Autodesk Fusion 360 part; units mm, degrees
(part 3 of 6)
  spline S37 degree 5 poles (53.0142, 47.6687) (53.0234, 47.6622) (53.0419, 47.6493) (53.0695, 47.6299) (53.1065, 47.6042) (53.1527, 47.5723) (53.1991, 47.5406) (53.2455, 47.5092) (53.292, 47.478) (53.3386, 47.4471) (53.3852, 47.4164) (53.4319, 47.3859) (53.4787, 47.3557) (53.5256, 47.3258) (53.5726, 47.2961) (53.6196, 47.2667) (53.6667, 47.2375) (53.7139, 47.2086) (53.7612, 47.1799) (53.8085, 47.1515) (53.8559, 47.1233) (53.9034, 47.0955) (53.951, 47.0679) (53.9986, 47.0405) (54.0463, 47.0135) (54.0941, 46.9867) (54.142, 46.9602) (54.1899, 46.9339) (54.2379, 46.908) (54.286, 46.8823) (54.3341, 46.8569) (54.3823, 46.8318) (54.4306, 46.807) (54.4789, 46.7825) (54.5273, 46.7583) (54.5758, 46.7344) (54.6244, 46.7108) (54.673, 46.6875) (54.7217, 46.6646) (54.7704, 46.6419) (54.8193, 46.6196) (54.8682, 46.5976) (54.9171, 46.5759) (54.9662, 46.5546) (55.0152, 46.5336) (55.0644, 46.5129) (55.1136, 46.4926) (55.1629, 46.4726) (55.2123, 46.453) (55.2617, 46.4338) (55.3112, 46.4149) (55.3607, 46.3965) (55.4103, 46.3784) (55.46, 46.3608) (55.5098, 46.3436) (55.5596, 46.3268) (55.6095, 46.3104) (55.6594, 46.2943) (55.7094, 46.2787) (55.7594, 46.2635) (55.8095, 46.2488) (55.8597, 46.2348) (55.91, 46.2215) (55.9604, 46.2089) (56.0108, 46.1968) (56.0613, 46.1852) (56.1118, 46.1739) (56.1624, 46.163) (56.213, 46.1525) (56.2636, 46.143) (56.3144, 46.1348) (56.3552, 46.1299) (56.3859, 46.1272) (56.4064, 46.126) (56.4167, 46.1255) knots -1 -1 -1 -1 -1 -1 -0.98571429 -0.97142857 -0.95714286 -0.94285714 -0.92857143 -0.91428571 -0.9 -0.88571429 -0.87142857 -0.85714286 -0.84285714 -0.82857143 -0.81428571 -0.8 -0.78571429 -0.77142857 -0.75714286 -0.74285714 -0.72857143 -0.71428571 -0.7 -0.68571429 -0.67142857 -0.65714286 -0.64285714 -0.62857143 -0.61428571 -0.6 -0.58571429 -0.57142857 -0.55714286 -0.54285714 -0.52857143 -0.51428571 -0.5 -0.48571429 -0.47142857 -0.45714286 -0.44285714 -0.42857143 -0.41428571 -0.4 -0.38571429 -0.37142857 -0.35714286 -0.34285714 -0.32857143 -0.31428571 -0.3 -0.28571429 -0.27142857 -0.25714286 -0.24285714 -0.22857143 -0.21428571 -0.2 -0.18571429 -0.17142857 -0.15714286 -0.14285714 -0.12857143 -0.11428571 -0.1 -0.08571429 -0.07142857 -0.05714286 -0.04285714 -0.02857143 -0.01428571 0 0 0 0 0 0
  line L37 (56.4167, 46.1255) -> (56.9142, 46.1012)
  arc A75 (57.3897, 45.5888) -> (56.9142, 46.1012) centre (56.8899, 45.6018) ccw
  arc A76 (57.3897, 45.5888) -> (57.3897, 44.4112) centre (79.882, 45) ccw
  arc A77 (56.9142, 43.8988) -> (57.3897, 44.4112) centre (56.8899, 44.3982) ccw
  line L38 (56.9142, 43.8988) -> (56.4167, 43.8745)
  spline S38 degree 5 poles (56.4167, 43.8745) (56.4064, 43.874) (56.3859, 43.8728) (56.3552, 43.8701) (56.3144, 43.8652) (56.2636, 43.857) (56.213, 43.8475) (56.1624, 43.837) (56.1118, 43.8261) (56.0613, 43.8148) (56.0108, 43.8032) (55.9604, 43.7911) (55.91, 43.7785) (55.8597, 43.7652) (55.8095, 43.7512) (55.7594, 43.7365) (55.7094, 43.7213) (55.6594, 43.7057) (55.6095, 43.6896) (55.5596, 43.6732) (55.5098, 43.6564) (55.46, 43.6392) (55.4103, 43.6216) (55.3607, 43.6035) (55.3112, 43.5851) (55.2617, 43.5662) (55.2123, 43.547) (55.1629, 43.5274) (55.1136, 43.5074) (55.0644, 43.4871) (55.0152, 43.4664) (54.9662, 43.4454) (54.9171, 43.4241) (54.8682, 43.4024) (54.8193, 43.3804) (54.7704, 43.3581) (54.7217, 43.3354) (54.673, 43.3125) (54.6244, 43.2892) (54.5758, 43.2656) (54.5273, 43.2417) (54.4789, 43.2175) (54.4306, 43.193) (54.3823, 43.1682) (54.3341, 43.1431) (54.286, 43.1177) (54.2379, 43.092) (54.1899, 43.0661) (54.142, 43.0398) (54.0941, 43.0133) (54.0463, 42.9865) (53.9986, 42.9595) (53.951, 42.9321) (53.9034, 42.9045) (53.8559, 42.8767) (53.8085, 42.8485) (53.7612, 42.8201) (53.7139, 42.7914) (53.6667, 42.7625) (53.6196, 42.7333) (53.5726, 42.7039) (53.5256, 42.6742) (53.4787, 42.6443) (53.4319, 42.6141) (53.3852, 42.5836) (53.3386, 42.5529) (53.292, 42.522) (53.2455, 42.4908) (53.1991, 42.4594) (53.1527, 42.4277) (53.1065, 42.3958) (53.0695, 42.3701) (53.0419, 42.3507) (53.0234, 42.3378) (53.0142, 42.3313) knots 0 0 0 0 0 0 0.01428571 0.02857143 0.04285714 0.05714286 0.07142857 0.08571429 0.1 0.11428571 0.12857143 0.14285714 0.15714286 0.17142857 0.18571429 0.2 0.21428571 0.22857143 0.24285714 0.25714286 0.27142857 0.28571429 0.3 0.31428571 0.32857143 0.34285714 0.35714286 0.37142857 0.38571429 0.4 0.41428571 0.42857143 0.44285714 0.45714286 0.47142857 0.48571429 0.5 0.51428571 0.52857143 0.54285714 0.55714286 0.57142857 0.58571429 0.6 0.61428571 0.62857143 0.64285714 0.65714286 0.67142857 0.68571429 0.7 0.71428571 0.72857143 0.74285714 0.75714286 0.77142857 0.78571429 0.8 0.81428571 0.82857143 0.84285714 0.85714286 0.87142857 0.88571429 0.9 0.91428571 0.92857143 0.94285714 0.95714286 0.97142857 0.98571429 1 1 1 1 1 1
  arc A78 (53.0142, 42.3313) -> (53.1946, 40.9031) centre (79.882, 45) ccw
  spline S39 degree 5 poles (53.1946, 40.9031) (53.2052, 40.8991) (53.2263, 40.8912) (53.2579, 40.8793) (53.3001, 40.8635) (53.3528, 40.8441) (53.4055, 40.825) (53.4583, 40.8061) (53.5111, 40.7875) (53.5639, 40.7691) (53.6167, 40.751) (53.6696, 40.7331) (53.7224, 40.7155) (53.7753, 40.6982) (53.8281, 40.6811) (53.881, 40.6643) (53.9339, 40.6477) (53.9868, 40.6314) (54.0397, 40.6154) (54.0926, 40.5997) (54.1455, 40.5842) (54.1985, 40.569) (54.2514, 40.5541) (54.3043, 40.5395) (54.3573, 40.5251) (54.4102, 40.5111) (54.4632, 40.4973) (54.5161, 40.4838) (54.569, 40.4706) (54.622, 40.4577) (54.6749, 40.4451) (54.7279, 40.4328) (54.7808, 40.4207) (54.8337, 40.409) (54.8866, 40.3976) (54.9395, 40.3865) (54.9924, 40.3758) (55.0453, 40.3653) (55.0982, 40.3552) (55.151, 40.3453) (55.2039, 40.3358) (55.2567, 40.3267) (55.3095, 40.3179) (55.3623, 40.3094) (55.4151, 40.3013) (55.4679, 40.2935) (55.5206, 40.2861) (55.5733, 40.279) (55.626, 40.2723) (55.6786, 40.2659) (55.7312, 40.2599) (55.7838, 40.2544) (55.8364, 40.2493) (55.8889, 40.2446) (55.9413, 40.2403) (55.9938, 40.2364) (56.0461, 40.2329) (56.0985, 40.2297) (56.1508, 40.227) (56.2031, 40.2247) (56.2552, 40.223) (56.3073, 40.2219) (56.3594, 40.2215) (56.4113, 40.2218) (56.4632, 40.2227) (56.5149, 40.224) (56.5667, 40.2256) (56.6183, 40.2276) (56.6699, 40.2301) (56.7214, 40.2334) (56.7726, 40.2381) (56.8133, 40.2435) (56.8437, 40.2486) (56.8639, 40.2525) (56.874, 40.2545) knots -1 -1 -1 -1 -1 -1 -0.98571429 -0.97142857 -0.95714286 -0.94285714 -0.92857143 -0.91428571 -0.9 -0.88571429 -0.87142857 -0.85714286 -0.84285714 -0.82857143 -0.81428571 -0.8 -0.78571429 -0.77142857 -0.75714286 -0.74285714 -0.72857143 -0.71428571 -0.7 -0.68571429 -0.67142857 -0.65714286 -0.64285714 -0.62857143 -0.61428571 -0.6 -0.58571429 -0.57142857 -0.55714286 -0.54285714 -0.52857143 -0.51428571 -0.5 -0.48571429 -0.47142857 -0.45714286 -0.44285714 -0.42857143 -0.41428571 -0.4 -0.38571429 -0.37142857 -0.35714286 -0.34285714 -0.32857143 -0.31428571 -0.3 -0.28571429 -0.27142857 -0.25714286 -0.24285714 -0.22857143 -0.21428571 -0.2 -0.18571429 -0.17142857 -0.15714286 -0.14285714 -0.12857143 -0.11428571 -0.1 -0.08571429 -0.07142857 -0.05714286 -0.04285714 -0.02857143 -0.01428571 0 0 0 0 0 0
  line L39 (56.874, 40.2545) -> (57.3619, 40.3548)
  arc A79 (57.9499, 39.9767) -> (57.3619, 40.3548) centre (57.4626, 39.865) ccw
  arc A80 (57.9499, 39.9767) -> (58.2428, 38.8361) centre (79.882, 45) ccw
  arc A81 (57.9097, 38.2215) -> (58.2428, 38.8361) centre (57.7619, 38.6992) ccw
  line L40 (57.9097, 38.2215) -> (57.4338, 38.0743)
  spline S40 degree 5 poles (57.4338, 38.0743) (57.424, 38.0712) (57.4044, 38.0649) (57.3753, 38.0547) (57.337, 38.0398) (57.2899, 38.0193) (57.2432, 37.9974) (57.1968, 37.9747) (57.1506, 37.9515) (57.1044, 37.9281) (57.0584, 37.9043) (57.0126, 37.88) (56.9669, 37.8553) (56.9215, 37.8299) (56.8764, 37.8038) (56.8315, 37.7772) (56.7868, 37.75) (56.7423, 37.7224) (56.6979, 37.6944) (56.6537, 37.6661) (56.6096, 37.6375) (56.5657, 37.6084) (56.522, 37.579) (56.4784, 37.5492) (56.435, 37.519) (56.3917, 37.4884) (56.3487, 37.4575) (56.3057, 37.4262) (56.263, 37.3946) (56.2203, 37.3627) (56.1779, 37.3305) (56.1355, 37.298) (56.0934, 37.2651) (56.0513, 37.2319) (56.0094, 37.1985) (55.9677, 37.1647) (55.9261, 37.1306) (55.8847, 37.0962) (55.8434, 37.0616) (55.8022, 37.0267) (55.7612, 36.9915) (55.7203, 36.956) (55.6796, 36.9202) (55.639, 36.8842) (55.5985, 36.8479) (55.5582, 36.8114) (55.518, 36.7745) (55.478, 36.7375) (55.4381, 36.7001) (55.3984, 36.6626) (55.3587, 36.6247) (55.3193, 36.5866) (55.2799, 36.5483) (55.2407, 36.5097) (55.2017, 36.4709) (55.1627, 36.4319) (55.1239, 36.3926) (55.0853, 36.3531) (55.0468, 36.3133) (55.0084, 36.2734) (54.9702, 36.2331) (54.9321, 36.1927) (54.8941, 36.152) (54.8563, 36.1112) (54.8186, 36.07) (54.781, 36.0287) (54.7436, 35.9872) (54.7063, 35.9454) (54.6692, 35.9034) (54.6322, 35.8613) (54.5953, 35.8189) (54.5659, 35.7848) (54.544, 35.7591) (54.5293, 35.7419) (54.522, 35.7334) knots 0 0 0 0 0 0 0.01428571 0.02857143 0.04285714 0.05714286 0.07142857 0.08571429 0.1 0.11428571 0.12857143 0.14285714 0.15714286 0.17142857 0.18571429 0.2 0.21428571 0.22857143 0.24285714 0.25714286 0.27142857 0.28571429 0.3 0.31428571 0.32857143 0.34285714 0.35714286 0.37142857 0.38571429 0.4 0.41428571 0.42857143 0.44285714 0.45714286 0.47142857 0.48571429 0.5 0.51428571 0.52857143 0.54285714 0.55714286 0.57142857 0.58571429 0.6 0.61428571 0.62857143 0.64285714 0.65714286 0.67142857 0.68571429 0.7 0.71428571 0.72857143 0.74285714 0.75714286 0.77142857 0.78571429 0.8 0.81428571 0.82857143 0.84285714 0.85714286 0.87142857 0.88571429 0.9 0.91428571 0.92857143 0.94285714 0.95714286 0.97142857 0.98571429 1 1 1 1 1 1
  arc A82 (54.522, 35.7334) -> (55.0519, 34.395) centre (79.882, 45) ccw
  spline S41 degree 5 poles (55.0519, 34.395) (55.0631, 34.3937) (55.0855, 34.3912) (55.1191, 34.3876) (55.1639, 34.3828) (55.2198, 34.3772) (55.2756, 34.3717) (55.3314, 34.3666) (55.3872, 34.3616) (55.4429, 34.357) (55.4986, 34.3526) (55.5542, 34.3484) (55.6098, 34.3445) (55.6653, 34.3408) (55.7207, 34.3374) (55.7761, 34.3343) (55.8315, 34.3314) (55.8868, 34.3288) (55.942, 34.3265) (55.9972, 34.3244) (56.0523, 34.3225) (56.1073, 34.321) (56.1623, 34.3197) (56.2172, 34.3187) (56.272, 34.318) (56.3268, 34.3175) (56.3815, 34.3173) (56.4362, 34.3174) (56.4907, 34.3178) (56.5452, 34.3185) (56.5996, 34.3194) (56.654, 34.3207) (56.7082, 34.3222) (56.7624, 34.324) (56.8165, 34.3261) (56.8705, 34.3285) (56.9244, 34.3313) (56.9782, 34.3343) (57.0319, 34.3376) (57.0856, 34.3412) (57.1391, 34.3452) (57.1926, 34.3494) (57.2459, 34.354) (57.2992, 34.359) (57.3523, 34.3642) (57.4053, 34.3698) (57.4582, 34.3757) (57.5111, 34.382) (57.5638, 34.3886) (57.6163, 34.3955) (57.6688, 34.4028) (57.7211, 34.4105) (57.7733, 34.4186) (57.8253, 34.4271) (57.8772, 34.436) (57.9289, 34.4453) (57.9805, 34.4549) (58.032, 34.4649) (58.0834, 34.4752) (58.1345, 34.486) (58.1855, 34.4974) (58.2362, 34.5093) (58.2867, 34.5218) (58.337, 34.535) (58.387, 34.5487) (58.4368, 34.5629) (58.4865, 34.5773) (58.5361, 34.5921) (58.5854, 34.6073) (58.6344, 34.6233) (58.6829, 34.6407) (58.721, 34.656) (58.7491, 34.6685) (58.7677, 34.6773) (58.777, 34.6818) knots -1 -1 -1 -1 -1 -1 -0.98571429 -0.97142857 -0.95714286 -0.94285714 -0.92857143 -0.91428571 -0.9 -0.88571429 -0.87142857 -0.85714286 -0.84285714 -0.82857143 -0.81428571 -0.8 -0.78571429 -0.77142857 -0.75714286 -0.74285714 -0.72857143 -0.71428571 -0.7 -0.68571429 -0.67142857 -0.65714286 -0.64285714 -0.62857143 -0.61428571 -0.6 -0.58571429 -0.57142857 -0.55714286 -0.54285714 -0.52857143 -0.51428571 -0.5 -0.48571429 -0.47142857 -0.45714286 -0.44285714 -0.42857143 -0.41428571 -0.4 -0.38571429 -0.37142857 -0.35714286 -0.34285714 -0.32857143 -0.31428571 -0.3 -0.28571429 -0.27142857 -0.25714286 -0.24285714 -0.22857143 -0.21428571 -0.2 -0.18571429 -0.17142857 -0.15714286 -0.14285714 -0.12857143 -0.11428571 -0.1 -0.08571429 -0.07142857 -0.05714286 -0.04285714 -0.02857143 -0.01428571 0 0 0 0 0 0
  line L41 (58.777, 34.6818) -> (59.2247, 34.9002)
  arc A83 (59.8882, 34.6802) -> (59.2247, 34.9002) centre (59.4439, 34.4509) ccw
  arc A84 (59.8882, 34.6802) -> (60.4555, 33.6483) centre (79.882, 45) ccw
  arc A85 (60.2857, 32.9702) -> (60.4555, 33.6483) centre (60.0238, 33.3961) ccw
  line L42 (60.2857, 32.9702) -> (59.8614, 32.7092)
  spline S42 degree 5 poles (59.8614, 32.7092) (59.8526, 32.7038) (59.8353, 32.6928) (59.8096, 32.6757) (59.7763, 32.6518) (59.7357, 32.6202) (59.6959, 32.5874) (59.6566, 32.5538) (59.6176, 32.5199) (59.5788, 32.4857) (59.5401, 32.4512) (59.5017, 32.4163) (59.4637, 32.381) (59.426, 32.3451) (59.3888, 32.3086) (59.3519, 32.2717) (59.3154, 32.2342) (59.2791, 32.1964) (59.2431, 32.1583) (59.2073, 32.1199) (59.1718, 32.0812) (59.1364, 32.0421) (59.1014, 32.0028) (59.0666, 31.9631) (59.0321, 31.923) (58.9978, 31.8826) (58.9638, 31.842) (58.93, 31.801) (58.8964, 31.7598) (58.863, 31.7182) (58.8299, 31.6765) (58.797, 31.6344) (58.7643, 31.5921) (58.7318, 31.5495) (58.6996, 31.5067) (58.6676, 31.4636) (58.6358, 31.4202) (58.6042, 31.3767) (58.5728, 31.3328) (58.5416, 31.2888) (58.5106, 31.2445) (58.4799, 31.1999) (58.4493, 31.1552) (58.4189, 31.1102) (58.3888, 31.065) (58.3588, 31.0195) (58.3291, 30.9739) (58.2995, 30.928) (58.2702, 30.8819) (58.241, 30.8356) (58.212, 30.7892) (58.1833, 30.7425) (58.1547, 30.6955) (58.1263, 30.6484) (58.0981, 30.6011) (58.0701, 30.5536) (58.0423, 30.5059) (58.0147, 30.4581) (57.9873, 30.41) (57.9601, 30.3617) (57.933, 30.3132) (57.9062, 30.2646) (57.8795, 30.2158) (57.8531, 30.1668) (57.8268, 30.1176) (57.8007, 30.0682) (57.7748, 30.0187) (57.7491, 29.9689) (57.7235, 29.9191) (57.6982, 29.869) (57.673, 29.8187) (57.653, 29.7784) (57.6381, 29.7481) (57.6282, 29.7278) (57.6233, 29.7177) knots 0 0 0 0 0 0 0.01428571 0.02857143 0.04285714 0.05714286 0.07142857 0.08571429 0.1 0.11428571 0.12857143 0.14285714 0.15714286 0.17142857 0.18571429 0.2 0.21428571 0.22857143 0.24285714 0.25714286 0.27142857 0.28571429 0.3 0.31428571 0.32857143 0.34285714 0.35714286 0.37142857 0.38571429 0.4 0.41428571 0.42857143 0.44285714 0.45714286 0.47142857 0.48571429 0.5 0.51428571 0.52857143 0.54285714 0.55714286 0.57142857 0.58571429 0.6 0.61428571 0.62857143 0.64285714 0.65714286 0.67142857 0.68571429 0.7 0.71428571 0.72857143 0.74285714 0.75714286 0.77142857 0.78571429 0.8 0.81428571 0.82857143 0.84285714 0.85714286 0.87142857 0.88571429 0.9 0.91428571 0.92857143 0.94285714 0.95714286 0.97142857 0.98571429 1 1 1 1 1 1
  arc A86 (57.6233, 29.7177) -> (58.4694, 28.5532) centre (79.882, 45) ccw
  spline S43 degree 5 poles (58.4694, 28.5532) (58.4805, 28.5547) (58.5028, 28.5579) (58.5363, 28.5627) (58.5808, 28.5692) (58.6364, 28.5776) (58.6918, 28.5863) (58.7472, 28.5952) (58.8024, 28.6043) (58.8575, 28.6136) (58.9125, 28.6231) (58.9675, 28.6329) (59.0222, 28.643) (59.0769, 28.6532) (59.1315, 28.6637) (59.1859, 28.6745) (59.2402, 28.6855) (59.2944, 28.6967) (59.3485, 28.7081) (59.4025, 28.7198) (59.4563, 28.7318) (59.51, 28.744) (59.5636, 28.7564) (59.617, 28.7691) (59.6703, 28.782) (59.7235, 28.7952) (59.7765, 28.8086) (59.8294, 28.8223) (59.8822, 28.8362) (59.9348, 28.8504) (59.9872, 28.8649) (60.0395, 28.8796) (60.0917, 28.8946) (60.1437, 28.9098) (60.1956, 28.9253) (60.2473, 28.9411) (60.2988, 28.9571) (60.3502, 28.9734) (60.4015, 28.99) (60.4525, 29.0069) (60.5034, 29.024) (60.5541, 29.0414) (60.6046, 29.0591) (60.655, 29.0771) (60.7051, 29.0955) (60.7551, 29.1141) (60.8049, 29.1329) (60.8545, 29.1521) (60.9039, 29.1716) (60.9531, 29.1914) (61.0021, 29.2115) (61.0508, 29.232) (61.0993, 29.2528) (61.1476, 29.274) (61.1957, 29.2955) (61.2435, 29.3174) (61.2911, 29.3395) (61.3384, 29.362) (61.3856, 29.3848) (61.4325, 29.408) (61.479, 29.4316) (61.5252, 29.4558) (61.571, 29.4805) (61.6164, 29.5057) (61.6614, 29.5315) (61.7061, 29.5576) (61.7507, 29.5839) (61.795, 29.6106) (61.839, 29.6376) (61.8825, 29.6653) (61.9251, 29.6941) (61.9582, 29.7184) (61.9824, 29.7375) (61.9982, 29.7507) (62.0061, 29.7573) knots -1 -1 -1 -1 -1 -1 -0.98571429 -0.97142857 -0.95714286 -0.94285714 -0.92857143 -0.91428571 -0.9 -0.88571429 -0.87142857 -0.85714286 -0.84285714 -0.82857143 -0.81428571 -0.8 -0.78571429 -0.77142857 -0.75714286 -0.74285714 -0.72857143 -0.71428571 -0.7 -0.68571429 -0.67142857 -0.65714286 -0.64285714 -0.62857143 -0.61428571 -0.6 -0.58571429 -0.57142857 -0.55714286 -0.54285714 -0.52857143 -0.51428571 -0.5 -0.48571429 -0.47142857 -0.45714286 -0.44285714 -0.42857143 -0.41428571 -0.4 -0.38571429 -0.37142857 -0.35714286 -0.34285714 -0.32857143 -0.31428571 -0.3 -0.28571429 -0.27142857 -0.25714286 -0.24285714 -0.22857143 -0.21428571 -0.2 -0.18571429 -0.17142857 -0.15714286 -0.14285714 -0.12857143 -0.11428571 -0.1 -0.08571429 -0.07142857 -0.05714286 -0.04285714 -0.02857143 -0.01428571 0 0 0 0 0 0
  line L43 (62.0061, 29.7573) -> (62.3854, 30.0802)
  arc A87 (63.0828, 30.0321) -> (62.3854, 30.0802) centre (62.7095, 29.6995) ccw
  arc A88 (63.0828, 30.0321) -> (63.8889, 29.1738) centre (79.882, 45) ccw
  arc A89 (63.8931, 28.4747) -> (63.8889, 29.1738) centre (63.5335, 28.8221) ccw
  line L44 (63.8931, 28.4747) -> (63.547, 28.1164)
  spline S44 degree 5 poles (63.547, 28.1164) (63.5398, 28.109) (63.5257, 28.0941) (63.5052, 28.0711) (63.4788, 28.0396) (63.4473, 27.9989) (63.417, 27.9573) (63.3873, 27.915) (63.3579, 27.8724) (63.3288, 27.8296) (63.2999, 27.7866) (63.2714, 27.7433) (63.2434, 27.6996) (63.2158, 27.6555) (63.1888, 27.6109) (63.1623, 27.5659) (63.1362, 27.5206) (63.1105, 27.4749) (63.0851, 27.4291) (63.06, 27.3829) (63.0352, 27.3366) (63.0107, 27.29) (62.9865, 27.2432) (62.9627, 27.196) (62.9392, 27.1487) (62.9161, 27.101) (62.8932, 27.0532) (62.8707, 27.0051) (62.8484, 26.9568) (62.8264, 26.9083) (62.8047, 26.8596) (62.7833, 26.8107) (62.7622, 26.7616) (62.7413, 26.7123) (62.7207, 26.6628) (62.7004, 26.613) (62.6804, 26.5632) (62.6606, 26.5131) (62.6411, 26.4628) (62.6219, 26.4124) (62.6029, 26.3618) (62.5842, 26.311) (62.5657, 26.26) (62.5475, 26.2089) (62.5295, 26.1576) (62.5118, 26.1062) (62.4943, 26.0545) (62.4771, 26.0028) (62.4601, 25.9508) (62.4434, 25.8987) (62.4269, 25.8465) (62.4107, 25.7941) (62.3947, 25.7416) (62.3789, 25.6889) (62.3634, 25.6361) (62.3481, 25.5831) (62.333, 25.53) (62.3182, 25.4767) (62.3036, 25.4234) (62.2892, 25.3698) (62.2751, 25.3162) (62.2612, 25.2624) (62.2475, 25.2085) (62.234, 25.1544) (62.2208, 25.1002) (62.2078, 25.0459) (62.195, 24.9915) (62.1825, 24.9369) (62.1701, 24.8823) (62.158, 24.8275) (62.1462, 24.7725) (62.1368, 24.7285) (62.1299, 24.6954) (62.1254, 24.6734) (62.1231, 24.6623) knots 0 0 0 0 0 0 0.01428571 0.02857143 0.04285714 0.05714286 0.07142857 0.08571429 0.1 0.11428571 0.12857143 0.14285714 0.15714286 0.17142857 0.18571429 0.2 0.21428571 0.22857143 0.24285714 0.25714286 0.27142857 0.28571429 0.3 0.31428571 0.32857143 0.34285714 0.35714286 0.37142857 0.38571429 0.4 0.41428571 0.42857143 0.44285714 0.45714286 0.47142857 0.48571429 0.5 0.51428571 0.52857143 0.54285714 0.55714286 0.57142857 0.58571429 0.6 0.61428571 0.62857143 0.64285714 0.65714286 0.67142857 0.68571429 0.7 0.71428571 0.72857143 0.74285714 0.75714286 0.77142857 0.78571429 0.8 0.81428571 0.82857143 0.84285714 0.85714286 0.87142857 0.88571429 0.9 0.91428571 0.92857143 0.94285714 0.95714286 0.97142857 0.98571429 1 1 1 1 1 1
  arc A90 (62.1231, 24.6623) -> (63.2322, 23.7448) centre (79.882, 45) ccw
  spline S45 degree 5 poles (63.2322, 23.7448) (63.2427, 23.7491) (63.2635, 23.7577) (63.2947, 23.7706) (63.3362, 23.788) (63.3879, 23.81) (63.4395, 23.8322) (63.4909, 23.8545) (63.5421, 23.8771) (63.5932, 23.8998) (63.6441, 23.9228) (63.6948, 23.9459) (63.7454, 23.9692) (63.7958, 23.9928) (63.8461, 24.0165) (63.8961, 24.0405) (63.946, 24.0646) (63.9957, 24.089) (64.0452, 24.1135) (64.0946, 24.1383) (64.1437, 24.1632) (64.1927, 24.1884) (64.2415, 24.2137) (64.2901, 24.2393) (64.3385, 24.2651) (64.3868, 24.2911) (64.4348, 24.3173) (64.4826, 24.3437) (64.5303, 24.3703) (64.5777, 24.3971) (64.6249, 24.4242) (64.6719, 24.4514) (64.7187, 24.4789) (64.7653, 24.5066) (64.8117, 24.5345) (64.8579, 24.5626) (64.9038, 24.591) (64.9495, 24.6196) (64.995, 24.6484) (65.0403, 24.6774) (65.0853, 24.7066) (65.1301, 24.7361) (65.1746, 24.7659) (65.2189, 24.7958) (65.2629, 24.826) (65.3067, 24.8565) (65.3502, 24.8871) (65.3935, 24.9181) (65.4365, 24.9492) (65.4792, 24.9806) (65.5216, 25.0123) (65.5638, 25.0442) (65.6056, 25.0765) (65.6471, 25.109) (65.6883, 25.1418) (65.7291, 25.1748) (65.7697, 25.2081) (65.81, 25.2417) (65.85, 25.2755) (65.8897, 25.3096) (65.9289, 25.3441) (65.9676, 25.379) (66.0058, 25.4143) (66.0435, 25.45) (66.0807, 25.4862) (66.1175, 25.5226) (66.1541, 25.5592) (66.1905, 25.596) (66.2264, 25.6331) (66.2616, 25.6707) (66.2957, 25.7093) (66.3217, 25.7411) (66.3404, 25.7656) (66.3524, 25.7822) (66.3584, 25.7906) knots -1 -1 -1 -1 -1 -1 -0.98571429 -0.97142857 -0.95714286 -0.94285714 -0.92857143 -0.91428571 -0.9 -0.88571429 -0.87142857 -0.85714286 -0.84285714 -0.82857143 -0.81428571 -0.8 -0.78571429 -0.77142857 -0.75714286 -0.74285714 -0.72857143 -0.71428571 -0.7 -0.68571429 -0.67142857 -0.65714286 -0.64285714 -0.62857143 -0.61428571 -0.6 -0.58571429 -0.57142857 -0.55714286 -0.54285714 -0.52857143 -0.51428571 -0.5 -0.48571429 -0.47142857 -0.45714286 -0.44285714 -0.42857143 -0.41428571 -0.4 -0.38571429 -0.37142857 -0.35714286 -0.34285714 -0.32857143 -0.31428571 -0.3 -0.28571429 -0.27142857 -0.25714286 -0.24285714 -0.22857143 -0.21428571 -0.2 -0.18571429 -0.17142857 -0.15714286 -0.14285714 -0.12857143 -0.11428571 -0.1 -0.08571429 -0.07142857 -0.05714286 -0.04285714 -0.02857143 -0.01428571 0 0 0 0 0 0
  line L45 (66.3584, 25.7906) -> (66.6454, 26.1977)
  arc A91 (67.3329, 26.3246) -> (66.6454, 26.1977) centre (67.0541, 25.9096) ccw
  arc A92 (67.3329, 26.3246) -> (68.3271, 25.6937) centre (79.882, 45) ccw
  arc A93 (68.5051, 25.0176) -> (68.3271, 25.6937) centre (68.0704, 25.2646) ccw
  line L46 (68.5051, 25.0176) -> (68.2589, 24.5845)
  spline S46 degree 5 poles (68.2589, 24.5845) (68.2539, 24.5755) (68.2439, 24.5576) (68.2297, 24.5302) (68.212, 24.4931) (68.1917, 24.4459) (68.1726, 24.398) (68.1543, 24.3497) (68.1365, 24.3011) (68.1189, 24.2525) (68.1017, 24.2036) (68.0848, 24.1546) (68.0685, 24.1053) (68.0528, 24.0557) (68.0378, 24.0058) (68.0233, 23.9556) (68.0093, 23.9052) (67.9957, 23.8546) (67.9825, 23.8039) (67.9697, 23.753) (67.9572, 23.7019) (67.945, 23.6507) (67.9333, 23.5993) (67.9219, 23.5477) (67.9109, 23.496) (67.9004, 23.4441) (67.8901, 23.3921) (67.8803, 23.3399) (67.8707, 23.2876) (67.8615, 23.2351) (67.8526, 23.1826) (67.844, 23.1299) (67.8357, 23.077) (67.8278, 23.0241) (67.8202, 22.971) (67.8129, 22.9178) (67.8059, 22.8645) (67.7992, 22.8111) (67.7928, 22.7576) (67.7867, 22.7039) (67.7809, 22.6502) (67.7754, 22.5963) (67.7702, 22.5424) (67.7652, 22.4883) (67.7606, 22.4342) (67.7562, 22.3799) (67.7522, 22.3256) (67.7484, 22.2712) (67.7448, 22.2167) (67.7416, 22.162) (67.7386, 22.1073) (67.7359, 22.0526) (67.7334, 21.9977) (67.7313, 21.9427) (67.7294, 21.8877) (67.7277, 21.8326) (67.7263, 21.7774) (67.7252, 21.7221) (67.7243, 21.6668) (67.7237, 21.6114) (67.7234, 21.5559) (67.7233, 21.5003) (67.7235, 21.4447) (67.7239, 21.389) (67.7245, 21.3332) (67.7254, 21.2774) (67.7266, 21.2215) (67.728, 21.1656) (67.7297, 21.1095) (67.7316, 21.0534) (67.7337, 20.9973) (67.7356, 20.9523) (67.7372, 20.9186) (67.7383, 20.8961) (67.7388, 20.8848) knots 0 0 0 0 0 0 0.01428571 0.02857143 0.04285714 0.05714286 0.07142857 0.08571429 0.1 0.11428571 0.12857143 0.14285714 0.15714286 0.17142857 0.18571429 0.2 0.21428571 0.22857143 0.24285714 0.25714286 0.27142857 0.28571429 0.3 0.31428571 0.32857143 0.34285714 0.35714286 0.37142857 0.38571429 0.4 0.41428571 0.42857143 0.44285714 0.45714286 0.47142857 0.48571429 0.5 0.51428571 0.52857143 0.54285714 0.55714286 0.57142857 0.58571429 0.6 0.61428571 0.62857143 0.64285714 0.65714286 0.67142857 0.68571429 0.7 0.71428571 0.72857143 0.74285714 0.75714286 0.77142857 0.78571429 0.8 0.81428571 0.82857143 0.84285714 0.85714286 0.87142857 0.88571429 0.9 0.91428571 0.92857143 0.94285714 0.95714286 0.97142857 0.98571429 1 1 1 1 1 1
  arc A94 (67.7388, 20.8848) -> (69.0413, 20.2719) centre (79.882, 45) ccw
  spline S47 degree 5 poles (69.0413, 20.2719) (69.0503, 20.2787) (69.0684, 20.2922) (69.0954, 20.3125) (69.1312, 20.3397) (69.1759, 20.3738) (69.2203, 20.4081) (69.2645, 20.4425) (69.3085, 20.4771) (69.3523, 20.5119) (69.3959, 20.5467) (69.4393, 20.5818) (69.4825, 20.617) (69.5255, 20.6523) (69.5682, 20.6878) (69.6108, 20.7234) (69.6531, 20.7592) (69.6952, 20.7952) (69.737, 20.8312) (69.7787, 20.8675) (69.8201, 20.9039) (69.8613, 20.9404) (69.9022, 20.9771) (69.943, 21.014) (69.9834, 21.051) (70.0237, 21.0882) (70.0637, 21.1255) (70.1034, 21.163) (70.143, 21.2006) (70.1822, 21.2384) (70.2212, 21.2763) (70.26, 21.3144) (70.2985, 21.3526) (70.3367, 21.3911) (70.3747, 21.4296) (70.4124, 21.4683) (70.4499, 21.5072) (70.487, 21.5463) (70.5239, 21.5855) (70.5606, 21.6249) (70.5969, 21.6644) (70.6329, 21.7041) (70.6687, 21.744) (70.7041, 21.784) (70.7392, 21.8242) (70.7741, 21.8646) (70.8086, 21.9051) (70.8428, 21.9458) (70.8767, 21.9867) (70.9103, 22.0277) (70.9435, 22.069) (70.9764, 22.1104) (71.0089, 22.152) (71.041, 22.1938) (71.0727, 22.2358) (71.1041, 22.278) (71.1351, 22.3204) (71.1658, 22.3629) (71.1962, 22.4056) (71.2261, 22.4485) (71.2555, 22.4916) (71.2843, 22.535) (71.3125, 22.5787) (71.3401, 22.6227) (71.3672, 22.667) (71.3938, 22.7114) (71.4202, 22.756) (71.4462, 22.8007) (71.4718, 22.8455) (71.4965, 22.8908) (71.5199, 22.9365) (71.5372, 22.9738) (71.5492, 23.0022) (71.5568, 23.0213) (71.5604, 23.0309) knots -1 -1 -1 -1 -1 -1 -0.98571429 -0.97142857 -0.95714286 -0.94285714 -0.92857143 -0.91428571 -0.9 -0.88571429 -0.87142857 -0.85714286 -0.84285714 -0.82857143 -0.81428571 -0.8 -0.78571429 -0.77142857 -0.75714286 -0.74285714 -0.72857143 -0.71428571 -0.7 -0.68571429 -0.67142857 -0.65714286 -0.64285714 -0.62857143 -0.61428571 -0.6 -0.58571429 -0.57142857 -0.55714286 -0.54285714 -0.52857143 -0.51428571 -0.5 -0.48571429 -0.47142857 -0.45714286 -0.44285714 -0.42857143 -0.41428571 -0.4 -0.38571429 -0.37142857 -0.35714286 -0.34285714 -0.32857143 -0.31428571 -0.3 -0.28571429 -0.27142857 -0.25714286 -0.24285714 -0.22857143 -0.21428571 -0.2 -0.18571429 -0.17142857 -0.15714286 -0.14285714 -0.12857143 -0.11428571 -0.1 -0.08571429 -0.07142857 -0.05714286 -0.04285714 -0.02857143 -0.01428571 0 0 0 0 0 0
  line L47 (71.5604, 23.0309) -> (71.7372, 23.4966)
  arc A95 (72.3716, 23.7905) -> (71.7372, 23.4966) centre (72.2047, 23.3192) ccw
  arc A96 (72.3716, 23.7905) -> (73.4915, 23.4266) centre (79.882, 45) ccw
  arc A97 (73.8319, 22.816) -> (73.4915, 23.4266) centre (73.3494, 22.9472) ccw
  line L48 (73.8319, 22.816) -> (73.7012, 22.3353)
  spline S48 degree 5 poles (73.7012, 22.3353) (73.6985, 22.3254) (73.6934, 22.3055) (73.6864, 22.2755) (73.6785, 22.2352) (73.6705, 22.1844) (73.664, 22.1332) (73.6583, 22.0819) (73.6531, 22.0304) (73.6482, 21.9789) (73.6436, 21.9273) (73.6395, 21.8756) (73.636, 21.8238) (73.6331, 21.7719) (73.6309, 21.7198) (73.6294, 21.6676) (73.6283, 21.6153) (73.6278, 21.5629) (73.6276, 21.5105) (73.6278, 21.458) (73.6284, 21.4054) (73.6294, 21.3528) (73.6308, 21.3001) (73.6326, 21.2473) (73.6349, 21.1945) (73.6375, 21.1416) (73.6406, 21.0887) (73.644, 21.0357) (73.6477, 20.9826) (73.6518, 20.9295) (73.6563, 20.8764) (73.6611, 20.8232) (73.6662, 20.77) (73.6717, 20.7167) (73.6775, 20.6634) (73.6837, 20.6101) (73.6901, 20.5567) (73.697, 20.5033) (73.7041, 20.4499) (73.7115, 20.3964) (73.7193, 20.3429) (73.7273, 20.2894) (73.7357, 20.2358) (73.7443, 20.1823) (73.7533, 20.1287) (73.7626, 20.075) (73.7721, 20.0214) (73.782, 19.9677) (73.7921, 19.914) (73.8026, 19.8603) (73.8133, 19.8066) (73.8243, 19.7529) (73.8355, 19.6991) (73.8471, 19.6454) (73.8589, 19.5916) (73.8711, 19.5378) (73.8834, 19.484) (73.8961, 19.4302) (73.909, 19.3764) (73.9222, 19.3225) (73.9357, 19.2687) (73.9494, 19.2149) (73.9634, 19.161) (73.9776, 19.1072) (73.9922, 19.0533) (74.0069, 18.9995) (74.022, 18.9456) (74.0372, 18.8918) (74.0528, 18.8379) (74.0686, 18.7841) (74.0846, 18.7302) (74.0977, 18.6871) (74.1076, 18.6548) (74.1142, 18.6333) (74.1175, 18.6225) knots 0 0 0 0 0 0 0.01428571 0.02857143 0.04285714 0.05714286 0.07142857 0.08571429 0.1 0.11428571 0.12857143 0.14285714 0.15714286 0.17142857 0.18571429 0.2 0.21428571 0.22857143 0.24285714 0.25714286 0.27142857 0.28571429 0.3 0.31428571 0.32857143 0.34285714 0.35714286 0.37142857 0.38571429 0.4 0.41428571 0.42857143 0.44285714 0.45714286 0.47142857 0.48571429 0.5 0.51428571 0.52857143 0.54285714 0.55714286 0.57142857 0.58571429 0.6 0.61428571 0.62857143 0.64285714 0.65714286 0.67142857 0.68571429 0.7 0.71428571 0.72857143 0.74285714 0.75714286 0.77142857 0.78571429 0.8 0.81428571 0.82857143 0.84285714 0.85714286 0.87142857 0.88571429 0.9 0.91428571 0.92857143 0.94285714 0.95714286 0.97142857 0.98571429 1 1 1 1 1 1
  arc A98 (74.1175, 18.6225) -> (75.5315, 18.3528) centre (79.882, 45) ccw
  spline S49 degree 5 poles (75.5315, 18.3528) (75.5386, 18.3616) (75.5527, 18.3792) (75.5738, 18.4056) (75.6017, 18.4408) (75.6365, 18.485) (75.671, 18.5292) (75.7053, 18.5736) (75.7393, 18.618) (75.7731, 18.6626) (75.8067, 18.7072) (75.84, 18.7519) (75.8731, 18.7967) (75.9059, 18.8417) (75.9385, 18.8867) (75.9708, 18.9318) (76.0029, 18.9769) (76.0347, 19.0222) (76.0663, 19.0676) (76.0976, 19.1131) (76.1287, 19.1586) (76.1595, 19.2043) (76.19, 19.25) (76.2203, 19.2958) (76.2503, 19.3417) (76.28, 19.3877) (76.3095, 19.4338) (76.3387, 19.48) (76.3676, 19.5263) (76.3962, 19.5726) (76.4246, 19.6191) (76.4527, 19.6656) (76.4804, 19.7122) (76.5079, 19.759) (76.5351, 19.8058) (76.562, 19.8526) (76.5886, 19.8996) (76.6149, 19.9467) (76.6409, 19.9938) (76.6666, 20.0411) (76.6919, 20.0884) (76.717, 20.1358) (76.7417, 20.1833) (76.766, 20.2309) (76.7901, 20.2786) (76.8138, 20.3264) (76.8371, 20.3742) (76.8602, 20.4221) (76.8828, 20.4702) (76.9051, 20.5183) (76.9271, 20.5665) (76.9486, 20.6148) (76.9697, 20.6632) (76.9904, 20.7116) (77.0107, 20.7602) (77.0306, 20.8089) (77.0501, 20.8576) (77.0693, 20.9064) (77.0881, 20.9553) (77.1064, 21.0043) (77.1241, 21.0534) (77.1413, 21.1027) (77.1577, 21.152) (77.1735, 21.2015) (77.1887, 21.2511) (77.2034, 21.3007) (77.2179, 21.3504) (77.232, 21.4002) (77.2456, 21.45) (77.2583, 21.5) (77.2696, 21.5501) (77.2771, 21.5905) (77.2817, 21.621) (77.2842, 21.6414) (77.2853, 21.6516) knots -1 -1 -1 -1 -1 -1 -0.98571429 -0.97142857 -0.95714286 -0.94285714 -0.92857143 -0.91428571 -0.9 -0.88571429 -0.87142857 -0.85714286 -0.84285714 -0.82857143 -0.81428571 -0.8 -0.78571429 -0.77142857 -0.75714286 -0.74285714 -0.72857143 -0.71428571 -0.7 -0.68571429 -0.67142857 -0.65714286 -0.64285714 -0.62857143 -0.61428571 -0.6 -0.58571429 -0.57142857 -0.55714286 -0.54285714 -0.52857143 -0.51428571 -0.5 -0.48571429 -0.47142857 -0.45714286 -0.44285714 -0.42857143 -0.41428571 -0.4 -0.38571429 -0.37142857 -0.35714286 -0.34285714 -0.32857143 -0.31428571 -0.3 -0.28571429 -0.27142857 -0.25714286 -0.24285714 -0.22857143 -0.21428571 -0.2 -0.18571429 -0.17142857 -0.15714286 -0.14285714 -0.12857143 -0.11428571 -0.1 -0.08571429 -0.07142857 -0.05714286 -0.04285714 -0.02857143 -0.01428571 0 0 0 0 0 0
  line L49 (77.2853, 21.6516) -> (77.3408, 22.1467)
  arc A99 (77.8821, 22.5891) -> (77.3408, 22.1467) centre (77.8377, 22.091) ccw
  line L50 (79.882, 45) -> (99.5642, 63.4828) construction
  line L51 (94.2241, 62.3365) -> (103.1265, 70.6965)
  line L52 (106.9873, 66.5851) -> (98.0849, 58.2252)
  circle A100 centre (110.7338, 73.9718) radius 1.75
  arc A101 (111.7668, 69.0797) -> (105.9162, 75.3099) centre (110.7338, 73.9718) ccw
  arc A102 (103.1265, 70.6965) -> (105.9162, 75.3099) centre (96.281, 77.9862) ccw
  arc A103 (111.7668, 69.0797) -> (106.9873, 66.5851) centre (113.8328, 59.2954) ccw
  circle A104 centre (79.882, 45) radius 0.5
  circle A105 centre (79.882, 45) radius 1.75
  dimension "d193" = 3.5
  dimension "d194" = 10
  dimension "d195" = 10
  dimension "d1" = 3.5
  constraint coincident A0.centre A2.centre
  constraint midpoint A38 L50.end
  constraint midpoint A40 L51.start
  constraint midpoint A36 L52.end
  constraint parallel L50 L51
  constraint parallel L50 L52
  constraint concentric A100 A101
  constraint tangent L51 A102
  constraint tangent A101 A102
  constraint tangent A101 A103
  constraint tangent L52 A103
  constraint equal A102 A103
  measures "d193" diameter of A100
  measures "d194" diameter of A101
  measures "d195" radius of A102
  measures "d1" diameter of A105
extrude "Extruir4" add sketch "Boceto5" against normal up to surface (3 mm away) contours A36 A37 L18 S18 A38 S19 L19 A39 A40 L51 L52 A101 A102 A103
extrude "Extruir5" cut sketch "Boceto5" against normal up to surface (3 mm away) contours A105
sketch "Boceto6" plane through (3, 0, 0) normal (1, 0, 0) x (0, 1, 0)
  circle A0 centre (79.882, 45) radius 1.75
  circle A1 centre (110.7338, 73.9718) radius 1.75
  arc A2 (77.8821, 22.5891) -> (79.0573, 22.5151) centre (79.882, 45) ccw
  arc A3 (79.5389, 22.0084) -> (79.0573, 22.5151) centre (79.039, 22.0155) ccw
  line L0 (79.5389, 22.0084) -> (79.5319, 21.5103)
  spline S0 degree 5 poles (79.5319, 21.5103) (79.5317, 21.5) (79.5317, 21.4795) (79.5324, 21.4487) (79.5348, 21.4076) (79.5397, 21.3564) (79.5461, 21.3053) (79.5533, 21.2541) (79.5611, 21.203) (79.5692, 21.1519) (79.5776, 21.1008) (79.5864, 21.0497) (79.5959, 20.9986) (79.606, 20.9476) (79.6169, 20.8966) (79.6283, 20.8457) (79.6404, 20.7948) (79.6528, 20.7439) (79.6657, 20.6931) (79.679, 20.6423) (79.6926, 20.5915) (79.7067, 20.5408) (79.7211, 20.4901) (79.736, 20.4394) (79.7513, 20.3888) (79.767, 20.3382) (79.7831, 20.2877) (79.7996, 20.2372) (79.8165, 20.1868) (79.8336, 20.1364) (79.8512, 20.086) (79.869, 20.0357) (79.8872, 19.9854) (79.9058, 19.9352) (79.9247, 19.885) (79.9439, 19.8349) (79.9635, 19.7848) (79.9833, 19.7348) (80.0035, 19.6848) (80.024, 19.6348) (80.0448, 19.5849) (80.066, 19.5351) (80.0874, 19.4853) (80.1091, 19.4356) (80.1311, 19.3859) (80.1534, 19.3363) (80.176, 19.2867) (80.1989, 19.2371) (80.2221, 19.1877) (80.2455, 19.1382) (80.2693, 19.0889) (80.2933, 19.0396) (80.3176, 18.9903) (80.3421, 18.9411) (80.367, 18.892) (80.3921, 18.8429) (80.4175, 18.7938) (80.4431, 18.7449) (80.469, 18.696) (80.4952, 18.6471) (80.5216, 18.5983) (80.5483, 18.5496) (80.5752, 18.5009) (80.6024, 18.4523) (80.6299, 18.4038) (80.6576, 18.3553) (80.6855, 18.3068) (80.7137, 18.2585) (80.7422, 18.2102) (80.7709, 18.162) (80.7998, 18.1138) (80.8231, 18.0753) (80.8407, 18.0465) (80.8525, 18.0273) (80.8584, 18.0177) knots 0 0 0 0 0 0 0.01428571 0.02857143 0.04285714 0.05714286 0.07142857 0.08571429 0.1 0.11428571 0.12857143 0.14285714 0.15714286 0.17142857 0.18571429 0.2 0.21428571 0.22857143 0.24285714 0.25714286 0.27142857 0.28571429 0.3 0.31428571 0.32857143 0.34285714 0.35714286 0.37142857 0.38571429 0.4 0.41428571 0.42857143 0.44285714 0.45714286 0.47142857 0.48571429 0.5 0.51428571 0.52857143 0.54285714 0.55714286 0.57142857 0.58571429 0.6 0.61428571 0.62857143 0.64285714 0.65714286 0.67142857 0.68571429 0.7 0.71428571 0.72857143 0.74285714 0.75714286 0.77142857 0.78571429 0.8 0.81428571 0.82857143 0.84285714 0.85714286 0.87142857 0.88571429 0.9 0.91428571 0.92857143 0.94285714 0.95714286 0.97142857 0.98571429 1 1 1 1 1 1
  arc A4 (80.8584, 18.0177) -> (82.2951, 18.108) centre (79.882, 45) ccw
  spline S1 degree 5 poles (82.2951, 18.108) (82.2997, 18.1183) (82.309, 18.1388) (82.3229, 18.1697) (82.3412, 18.2108) (82.3639, 18.2622) (82.3863, 18.3136) (82.4085, 18.3651) (82.4304, 18.4166) (82.452, 18.4682) (82.4734, 18.5197) (82.4946, 18.5713) (82.5155, 18.623) (82.5361, 18.6746) (82.5565, 18.7263) (82.5766, 18.7781) (82.5964, 18.8298) (82.616, 18.8816) (82.6353, 18.9334) (82.6543, 18.9852) (82.6731, 19.037) (82.6916, 19.0889) (82.7098, 19.1408) (82.7277, 19.1927) (82.7453, 19.2447) (82.7627, 19.2966) (82.7798, 19.3486) (82.7966, 19.4006) (82.8131, 19.4526) (82.8293, 19.5046) (82.8452, 19.5566) (82.8608, 19.6087) (82.8761, 19.6608) (82.8911, 19.7129) (82.9058, 19.7649) (82.9202, 19.8171) (82.9343, 19.8692) (82.9481, 19.9213) (82.9615, 19.9734) (82.9746, 20.0256) (82.9874, 20.0777) (82.9999, 20.1299) (83.012, 20.182) (83.0238, 20.2342) (83.0352, 20.2863) (83.0462, 20.3385) (83.057, 20.3906) (83.0674, 20.4428) (83.0774, 20.495) (83.087, 20.5471) (83.0963, 20.5992) (83.1051, 20.6514) (83.1135, 20.7035) (83.1215, 20.7556) (83.1291, 20.8077) (83.1363, 20.8598) (83.1431, 20.9118) (83.1495, 20.9639) (83.1555, 21.0159) (83.161, 21.0679) (83.166, 21.1199) (83.1704, 21.1718) (83.174, 21.2237) (83.177, 21.2756) (83.1794, 21.3274) (83.1814, 21.3791) (83.183, 21.4309) (83.1842, 21.4826) (83.185, 21.5342) (83.1849, 21.5858) (83.1834, 21.6372) (83.1806, 21.6782) (83.1775, 21.7088) (83.1749, 21.7292) (83.1734, 21.7394) knots -1 -1 -1 -1 -1 -1 -0.98571429 -0.97142857 -0.95714286 -0.94285714 -0.92857143 -0.91428571 -0.9 -0.88571429 -0.87142857 -0.85714286 -0.84285714 -0.82857143 -0.81428571 -0.8 -0.78571429 -0.77142857 -0.75714286 -0.74285714 -0.72857143 -0.71428571 -0.7 -0.68571429 -0.67142857 -0.65714286 -0.64285714 -0.62857143 -0.61428571 -0.6 -0.58571429 -0.57142857 -0.55714286 -0.54285714 -0.52857143 -0.51428571 -0.5 -0.48571429 -0.47142857 -0.45714286 -0.44285714 -0.42857143 -0.41428571 -0.4 -0.38571429 -0.37142857 -0.35714286 -0.34285714 -0.32857143 -0.31428571 -0.3 -0.28571429 -0.27142857 -0.25714286 -0.24285714 -0.22857143 -0.21428571 -0.2 -0.18571429 -0.17142857 -0.15714286 -0.14285714 -0.12857143 -0.11428571 -0.1 -0.08571429 -0.07142857 -0.05714286 -0.04285714 -0.02857143 -0.01428571 0 0 0 0 0 0
  line L1 (83.1734, 21.7394) -> (83.104, 22.2327)
  arc A5 (83.5183, 22.7958) -> (83.104, 22.2327) centre (83.5991, 22.3024) ccw
  arc A6 (83.5183, 22.7958) -> (84.675, 23.0164) centre (79.882, 45) ccw
  arc A7 (85.2675, 22.6454) -> (84.675, 23.0164) centre (84.7815, 22.5279) ccw
  line L2 (85.2675, 22.6454) -> (85.3845, 22.1612)
  spline S2 degree 5 poles (85.3845, 22.1612) (85.387, 22.1512) (85.392, 22.1313) (85.4004, 22.1016) (85.4129, 22.0625) (85.4304, 22.0141) (85.4493, 21.9661) (85.469, 21.9184) (85.4892, 21.8708) (85.5098, 21.8233) (85.5306, 21.7759) (85.5519, 21.7286) (85.5738, 21.6815) (85.5963, 21.6346) (85.6195, 21.5879) (85.6432, 21.5414) (85.6675, 21.4951) (85.6923, 21.449) (85.7174, 21.4029) (85.7429, 21.357) (85.7687, 21.3112) (85.7949, 21.2656) (85.8216, 21.2201) (85.8486, 21.1747) (85.876, 21.1295) (85.9038, 21.0844) (85.932, 21.0395) (85.9605, 20.9947) (85.9893, 20.95) (86.0185, 20.9055) (86.048, 20.8611) (86.0778, 20.8168) (86.108, 20.7726) (86.1384, 20.7286) (86.1692, 20.6847) (86.2003, 20.6409) (86.2317, 20.5972) (86.2634, 20.5537) (86.2954, 20.5103) (86.3276, 20.467) (86.3602, 20.4239) (86.393, 20.3809) (86.4262, 20.338) (86.4596, 20.2952) (86.4932, 20.2525) (86.5272, 20.21) (86.5614, 20.1676) (86.5959, 20.1253) (86.6307, 20.0832) (86.6657, 20.0411) (86.7009, 19.9992) (86.7365, 19.9574) (86.7722, 19.9158) (86.8083, 19.8742) (86.8446, 19.8328) (86.8811, 19.7915) (86.9179, 19.7503) (86.9549, 19.7093) (86.9921, 19.6683) (87.0296, 19.6275) (87.0673, 19.5868) (87.1053, 19.5463) (87.1435, 19.5058) (87.1819, 19.4655) (87.2206, 19.4253) (87.2595, 19.3852) (87.2986, 19.3453) (87.3379, 19.3055) (87.3775, 19.2657) (87.4173, 19.2262) (87.4573, 19.1867) (87.4895, 19.1552) (87.5137, 19.1317) (87.5299, 19.116) (87.538, 19.1082) knots 0 0 0 0 0 0 0.01428571 0.02857143 0.04285714 0.05714286 0.07142857 0.08571429 0.1 0.11428571 0.12857143 0.14285714 0.15714286 0.17142857 0.18571429 0.2 0.21428571 0.22857143 0.24285714 0.25714286 0.27142857 0.28571429 0.3 0.31428571 0.32857143 0.34285714 0.35714286 0.37142857 0.38571429 0.4 0.41428571 0.42857143 0.44285714 0.45714286 0.47142857 0.48571429 0.5 0.51428571 0.52857143 0.54285714 0.55714286 0.57142857 0.58571429 0.6 0.61428571 0.62857143 0.64285714 0.65714286 0.67142857 0.68571429 0.7 0.71428571 0.72857143 0.74285714 0.75714286 0.77142857 0.78571429 0.8 0.81428571 0.82857143 0.84285714 0.85714286 0.87142857 0.88571429 0.9 0.91428571 0.92857143 0.94285714 0.95714286 0.97142857 0.98571429 1 1 1 1 1 1
  arc A8 (87.538, 19.1082) -> (88.907, 19.553) centre (79.882, 45) ccw
  spline S3 degree 5 poles (88.907, 19.553) (88.909, 19.5641) (88.9129, 19.5863) (88.9186, 19.6196) (88.9262, 19.664) (88.9353, 19.7194) (88.9443, 19.7748) (88.9529, 19.8302) (88.9613, 19.8855) (88.9695, 19.9408) (88.9774, 19.9961) (88.9851, 20.0514) (88.9924, 20.1066) (88.9996, 20.1618) (89.0064, 20.2169) (89.0131, 20.272) (89.0194, 20.327) (89.0255, 20.382) (89.0313, 20.437) (89.0368, 20.4919) (89.0421, 20.5468) (89.0471, 20.6017) (89.0518, 20.6565) (89.0563, 20.7112) (89.0605, 20.7659) (89.0644, 20.8205) (89.068, 20.8751) (89.0713, 20.9296) (89.0744, 20.9841) (89.0771, 21.0385) (89.0796, 21.0929) (89.0818, 21.1472) (89.0837, 21.2015) (89.0852, 21.2556) (89.0865, 21.3097) (89.0875, 21.3638) (89.0882, 21.4178) (89.0886, 21.4717) (89.0886, 21.5255) (89.0884, 21.5793) (89.0878, 21.633) (89.0869, 21.6866) (89.0856, 21.7401) (89.0841, 21.7936) (89.0822, 21.8469) (89.0799, 21.9002) (89.0773, 21.9534) (89.0744, 22.0065) (89.0711, 22.0595) (89.0675, 22.1124) (89.0635, 22.1652) (89.0591, 22.2179) (89.0543, 22.2705) (89.0491, 22.3229) (89.0435, 22.3753) (89.0375, 22.4275) (89.0311, 22.4796) (89.0244, 22.5316) (89.0173, 22.5835) (89.0097, 22.6353) (89.0016, 22.6868) (88.9929, 22.7382) (88.9835, 22.7894) (88.9735, 22.8404) (88.963, 22.8911) (88.952, 22.9418) (88.9407, 22.9923) (88.929, 23.0427) (88.917, 23.0929) (88.9041, 23.1428) (88.8898, 23.1922) (88.8769, 23.2312) (88.8662, 23.2601) (88.8586, 23.2792) (88.8547, 23.2887) knots -1 -1 -1 -1 -1 -1 -0.98571429 -0.97142857 -0.95714286 -0.94285714 -0.92857143 -0.91428571 -0.9 -0.88571429 -0.87142857 -0.85714286 -0.84285714 -0.82857143 -0.81428571 -0.8 -0.78571429 -0.77142857 -0.75714286 -0.74285714 -0.72857143 -0.71428571 -0.7 -0.68571429 -0.67142857 -0.65714286 -0.64285714 -0.62857143 -0.61428571 -0.6 -0.58571429 -0.57142857 -0.55714286 -0.54285714 -0.52857143 -0.51428571 -0.5 -0.48571429 -0.47142857 -0.45714286 -0.44285714 -0.42857143 -0.41428571 -0.4 -0.38571429 -0.37142857 -0.35714286 -0.34285714 -0.32857143 -0.31428571 -0.3 -0.28571429 -0.27142857 -0.25714286 -0.24285714 -0.22857143 -0.21428571 -0.2 -0.18571429 -0.17142857 -0.15714286 -0.14285714 -0.12857143 -0.11428571 -0.1 -0.08571429 -0.07142857 -0.05714286 -0.04285714 -0.02857143 -0.01428571 0 0 0 0 0 0
  line L3 (88.8547, 23.2887) -> (88.6648, 23.7492)
  arc A9 (88.926, 24.3977) -> (88.6648, 23.7492) centre (89.127, 23.9399) ccw
  arc A10 (88.926, 24.3977) -> (89.9915, 24.899) centre (79.882, 45) ccw
  arc A11 (90.6577, 24.687) -> (89.9915, 24.899) centre (90.2161, 24.4524) ccw
  line L4 (90.6577, 24.687) -> (90.8915, 24.2471)
  spline S4 degree 5 poles (90.8915, 24.2471) (90.8963, 24.2381) (90.9061, 24.22) (90.9216, 24.1934) (90.9434, 24.1586) (90.9724, 24.1161) (91.0027, 24.0743) (91.0336, 24.033) (91.0651, 23.9919) (91.0968, 23.951) (91.1288, 23.9103) (91.1612, 23.8698) (91.194, 23.8296) (91.2275, 23.7898) (91.2616, 23.7503) (91.2961, 23.7112) (91.3312, 23.6724) (91.3667, 23.6338) (91.4024, 23.5955) (91.4385, 23.5573) (91.4749, 23.5194) (91.5117, 23.4817) (91.5488, 23.4443) (91.5862, 23.4071) (91.624, 23.3701) (91.6622, 23.3333) (91.7006, 23.2968) (91.7394, 23.2605) (91.7784, 23.2244) (91.8178, 23.1885) (91.8574, 23.1528) (91.8973, 23.1174) (91.9375, 23.0821) (91.9779, 23.047) (92.0186, 23.0121) (92.0596, 22.9775) (92.1009, 22.943) (92.1424, 22.9087) (92.1842, 22.8746) (92.2262, 22.8408) (92.2685, 22.8071) (92.311, 22.7736) (92.3538, 22.7402) (92.3968, 22.7071) (92.44, 22.6742) (92.4834, 22.6414) (92.5271, 22.6089) (92.5711, 22.5765) (92.6152, 22.5443) (92.6596, 22.5123) (92.7042, 22.4805) (92.749, 22.4488) (92.794, 22.4174) (92.8392, 22.3861) (92.8846, 22.355) (92.9303, 22.3241) (92.9761, 22.2933) (93.0222, 22.2628) (93.0685, 22.2324) (93.1149, 22.2022) (93.1616, 22.1722) (93.2085, 22.1423) (93.2555, 22.1126) (93.3028, 22.0831) (93.3502, 22.0538) (93.3978, 22.0247) (93.4457, 21.9957) (93.4937, 21.9669) (93.5419, 21.9383) (93.5902, 21.9098) (93.6388, 21.8816) (93.6778, 21.8591) (93.7071, 21.8423) (93.7267, 21.8312) (93.7365, 21.8256) knots 0 0 0 0 0 0 0.01428571 0.02857143 0.04285714 0.05714286 0.07142857 0.08571429 0.1 0.11428571 0.12857143 0.14285714 0.15714286 0.17142857 0.18571429 0.2 0.21428571 0.22857143 0.24285714 0.25714286 0.27142857 0.28571429 0.3 0.31428571 0.32857143 0.34285714 0.35714286 0.37142857 0.38571429 0.4 0.41428571 0.42857143 0.44285714 0.45714286 0.47142857 0.48571429 0.5 0.51428571 0.52857143 0.54285714 0.55714286 0.57142857 0.58571429 0.6 0.61428571 0.62857143 0.64285714 0.65714286 0.67142857 0.68571429 0.7 0.71428571 0.72857143 0.74285714 0.75714286 0.77142857 0.78571429 0.8 0.81428571 0.82857143 0.84285714 0.85714286 0.87142857 0.88571429 0.9 0.91428571 0.92857143 0.94285714 0.95714286 0.97142857 0.98571429 1 1 1 1 1 1
  arc A12 (93.7365, 21.8256) -> (94.9519, 22.5969) centre (79.882, 45) ccw
  spline S5 degree 5 poles (94.9519, 22.5969) (94.951, 22.6081) (94.9493, 22.6306) (94.9466, 22.6643) (94.9428, 22.7091) (94.9379, 22.7651) (94.9328, 22.821) (94.9274, 22.8768) (94.9218, 22.9325) (94.916, 22.9881) (94.9099, 23.0436) (94.9035, 23.099) (94.897, 23.1543) (94.8902, 23.2095) (94.8831, 23.2646) (94.8758, 23.3197) (94.8683, 23.3746) (94.8605, 23.4294) (94.8524, 23.484) (94.8441, 23.5386) (94.8356, 23.5931) (94.8268, 23.6475) (94.8178, 23.7017) (94.8085, 23.7558) (94.7989, 23.8098) (94.7891, 23.8637) (94.779, 23.9175) (94.7687, 23.9711) (94.7581, 24.0247) (94.7472, 24.0781) (94.7361, 24.1313) (94.7247, 24.1845) (94.713, 24.2375) (94.7011, 24.2904) (94.6889, 24.3431) (94.6764, 24.3957) (94.6636, 24.4481) (94.6506, 24.5004) (94.6372, 24.5526) (94.6236, 24.6046) (94.6097, 24.6565) (94.5955, 24.7082) (94.581, 24.7597) (94.5662, 24.8111) (94.5511, 24.8623) (94.5356, 24.9133) (94.5199, 24.9642) (94.5039, 25.0149) (94.4875, 25.0654) (94.4709, 25.1158) (94.4539, 25.1659) (94.4365, 25.2159) (94.4188, 25.2656) (94.4007, 25.3151) (94.3822, 25.3644) (94.3634, 25.4135) (94.3443, 25.4624) (94.3248, 25.5111) (94.305, 25.5596) (94.2848, 25.6078) (94.2642, 25.6558) (94.2429, 25.7034) (94.2212, 25.7506) (94.1988, 25.7975) (94.1759, 25.8441) (94.1527, 25.8904) (94.1292, 25.9365) (94.1054, 25.9824) (94.0812, 26.028) (94.0563, 26.0732) (94.0302, 26.1175) (94.008, 26.1521) (93.9905, 26.1774) (93.9783, 26.194) (93.9722, 26.2022) knots -1 -1 -1 -1 -1 -1 -0.98571429 -0.97142857 -0.95714286 -0.94285714 -0.92857143 -0.91428571 -0.9 -0.88571429 -0.87142857 -0.85714286 -0.84285714 -0.82857143 -0.81428571 -0.8 -0.78571429 -0.77142857 -0.75714286 -0.74285714 -0.72857143 -0.71428571 -0.7 -0.68571429 -0.67142857 -0.65714286 -0.64285714 -0.62857143 -0.61428571 -0.6 -0.58571429 -0.57142857 -0.55714286 -0.54285714 -0.52857143 -0.51428571 -0.5 -0.48571429 -0.47142857 -0.45714286 -0.44285714 -0.42857143 -0.41428571 -0.4 -0.38571429 -0.37142857 -0.35714286 -0.34285714 -0.32857143 -0.31428571 -0.3 -0.28571429 -0.27142857 -0.25714286 -0.24285714 -0.22857143 -0.21428571 -0.2 -0.18571429 -0.17142857 -0.15714286 -0.14285714 -0.12857143 -0.11428571 -0.1 -0.08571429 -0.07142857 -0.05714286 -0.04285714 -0.02857143 -0.01428571 0 0 0 0 0 0
  line L5 (93.9722, 26.2022) -> (93.6737, 26.6011)
  arc A13 (93.7655, 27.2941) -> (93.6737, 26.6011) centre (94.074, 26.9006) ccw
  arc A14 (93.7655, 27.2941) -> (94.6728, 28.0447) centre (79.882, 45) ccw
  arc A15 (95.3708, 28.005) -> (94.6728, 28.0447) centre (95.0015, 27.6679) ccw
  line L6 (95.3708, 28.005) -> (95.7066, 27.6371)
  spline S6 degree 5 poles (95.7066, 27.6371) (95.7135, 27.6295) (95.7276, 27.6145) (95.7492, 27.5925) (95.779, 27.5642) (95.8176, 27.5303) (95.8573, 27.4973) (95.8976, 27.465) (95.9382, 27.433) (95.9791, 27.4013) (96.0202, 27.3698) (96.0617, 27.3386) (96.1035, 27.3079) (96.1458, 27.2776) (96.1886, 27.2479) (96.2319, 27.2186) (96.2755, 27.1897) (96.3194, 27.1612) (96.3636, 27.1329) (96.408, 27.105) (96.4527, 27.0773) (96.4977, 27.0499) (96.5429, 27.0229) (96.5885, 26.9962) (96.6343, 26.9697) (96.6803, 26.9436) (96.7267, 26.9178) (96.7733, 26.8923) (96.8201, 26.8671) (96.8671, 26.8421) (96.9143, 26.8174) (96.9618, 26.7929) (97.0095, 26.7687) (97.0574, 26.7448) (97.1055, 26.7212) (97.1538, 26.6978) (97.2024, 26.6747) (97.2511, 26.6518) (97.3001, 26.6292) (97.3492, 26.6068) (97.3985, 26.5847) (97.448, 26.5628) (97.4977, 26.5412) (97.5476, 26.5198) (97.5977, 26.4986) (97.6479, 26.4777) (97.6983, 26.457) (97.7489, 26.4366) (97.7997, 26.4164) (97.8506, 26.3964) (97.9017, 26.3767) (97.953, 26.3572) (98.0044, 26.3379) (98.056, 26.3189) (98.1077, 26.3) (98.1596, 26.2814) (98.2117, 26.2631) (98.2639, 26.2449) (98.3163, 26.227) (98.3688, 26.2093) (98.4215, 26.1918) (98.4743, 26.1746) (98.5272, 26.1575) (98.5803, 26.1407) (98.6336, 26.1241) (98.687, 26.1077) (98.7405, 26.0916) (98.7941, 26.0756) (98.8479, 26.0599) (98.9019, 26.0444) (98.9559, 26.0291) (98.9993, 26.017) (99.0319, 26.008) (99.0536, 26.0021) (99.0645, 25.9991) knots 0 0 0 0 0 0 0.01428571 0.02857143 0.04285714 0.05714286 0.07142857 0.08571429 0.1 0.11428571 0.12857143 0.14285714 0.15714286 0.17142857 0.18571429 0.2 0.21428571 0.22857143 0.24285714 0.25714286 0.27142857 0.28571429 0.3 0.31428571 0.32857143 0.34285714 0.35714286 0.37142857 0.38571429 0.4 0.41428571 0.42857143 0.44285714 0.45714286 0.47142857 0.48571429 0.5 0.51428571 0.52857143 0.54285714 0.55714286 0.57142857 0.58571429 0.6 0.61428571 0.62857143 0.64285714 0.65714286 0.67142857 0.68571429 0.7 0.71428571 0.72857143 0.74285714 0.75714286 0.77142857 0.78571429 0.8 0.81428571 0.82857143 0.84285714 0.85714286 0.87142857 0.88571429 0.9 0.91428571 0.92857143 0.94285714 0.95714286 0.97142857 0.98571429 1 1 1 1 1 1
  arc A16 (99.0645, 25.9991) -> (100.0499, 27.0485) centre (79.882, 45) ccw